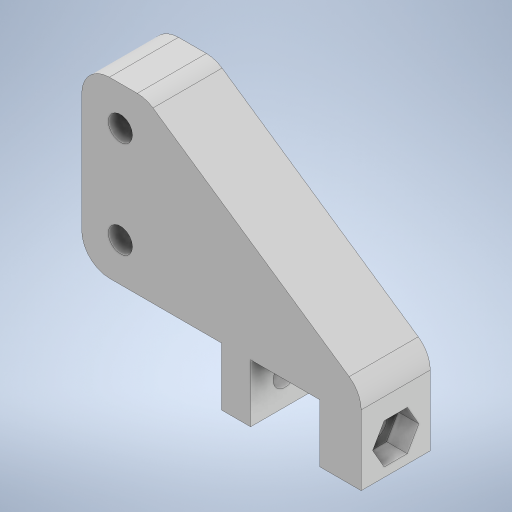
# Autodesk Inventor part: ClawShoulder
Saved by Autodesk Inventor 2023 (Build 270158000, 158)
## iProperties
Created: 2023-06-03
Part Number: ClawShoulder
Material: Ogólny
Document SubType Name: Modeling
Designer: Kamil
Density: 1 g/cm^3
Appearance: Domyślna
Author: Kamil
Autodesk Inventor part; units mm, degrees
ref_plane "YZ Plane" through (0, 0, 0) normal (1, 0, 0) x (0, 1, 0)
ref_plane "XZ Plane" through (0, 0, 0) normal (0, 1, 0) x (-1, 0, 0)
ref_plane "XY Plane" through (0, 0, 0) normal (0, 0, 1) x (1, 0, 0)
sketch "Szkic1" plane through (0, 0, 0) normal (0, 0, 1) x (1, 0, 0)
  line L0 (0.0002, 14.0002) -> (0.0002, 0.0002)
  line L1 (7.56, 19.5982) -> (5.6, 19.5982)
  line L2 (38.64, -14) -> (38.64, -5.6)
  line L3 (34.44, -14) -> (38.64, -14)
  line L4 (34.44, -5.6) -> (34.44, -14)
  line L5 (24.44, -14) -> (24.44, -5.6)
  line L6 (20.24, -14) -> (24.44, -14)
  line L7 (20.24, -5.6) -> (20.24, -14)
  circle A0 centre (5.6, 13.9982) radius 1.75
  circle A1 centre (5.6002, 0) radius 1.75
  line L8 (5.6, -5.6) -> (20.24, -5.6)
  line L9 (24.44, -5.6) -> (34.44, -5.6)
  line L10 (0, 19.5982) -> (9.2883, 19.5982)
  line L11 (0, -5.6) -> (0, 19.5982)
  line L12 (9.2883, 19.5982) -> (38.64, -0.5396)
  line L13 (38.64, -5.6) -> (38.64, -0.5396)
  line L14 (34.44, -5.6) -> (24.44, -5.6)
  line L15 (20.24, -5.6) -> (0, -5.6)
  point P0 (0, 0)
  point P1 (0, 14)
  point P2 (0, 0)
  dimension "d7" = 3.5
  dimension "d8" = 5.6
  dimension "d9" = 5.6
  dimension "d10" = 5.6
  dimension "d11" = 5.6
  dimension "d12" = 3.5
  constraints: 32 end point, 4 horizontal, 2 centre point, 2 parallel, 2 vertical, 1 other
  measures "d7" diameter of A0
  measures "d8" distance from line of L15 A1.centre
  measures "d9" distance from line of L11 A0.centre
  measures "d10" distance from line of L10 A0.centre
  measures "d11" distance from line of L0 A1.centre
  measures "d12" diameter of A1
extrude "Wyciągnięcie proste1" add sketch "Szkic1" against normal blind 10
sketch "Szkic2" plane through (20.24, -14, 0) normal (-1, 0, 0) x (0, 0, 1)
  line L0 (0, 8.4) -> (0, 0) projected
  line L1 (0, 8.4) -> (-10, 8.4) projected
  line L2 (-10, 0) -> (-10, 8.4) projected
  line L3 (0, 0) -> (-10, 0) projected
  line L4 (0, 0) -> (-10, 0) projected
  line L5 (-5, 0) -> (-5, 4.2)
  line L6 (-5, 4.2) -> (0, 4.2)
  circle A0 centre (-5, 4.2) radius 1.75
  point P0 (0, 14)
  dimension "d3" = 4.2
  dimension "d4" = 3.5
  constraints: 4 end point, 2 midpoint, 1 centre point, 1 coincident, 1 point on line, 1 vertical
  measures "d3" distance of L5.start L5.end
  measures "d4" diameter of A0
extrude "Wyciągnięcie proste2" cut sketch "Szkic2" against normal through all contours A0 L5 L6 | L6 L5 A0
move faces "Przesuń1" translate (1.8, 0, 0) faces at (38.64, -3.0473, -4.9297)
sketch "Szkic3" plane through (40.44, -14, 0) normal (1, 0, 0) x (0, 0, -1)
  circle A0 centre (5, 4.2) radius 1.75 projected
  circle A1 centre (5, 4.2) radius 2.9
  line L0 (3.3257, 1.3) -> (1.6514, 4.2)
  line L1 (1.6514, 4.2) -> (3.3257, 7.1)
  line L2 (3.3257, 7.1) -> (6.6743, 7.1)
  line L3 (6.6743, 7.1) -> (8.3486, 4.2)
  line L4 (8.3486, 4.2) -> (6.6743, 1.3)
  line L5 (6.6743, 1.3) -> (3.3257, 1.3)
  point P0 (0, 14)
  point P1 (5, 1.3)
  dimension "d16" = 5.8
  constraints: 12 end point, 2 coincident, 1 midpoint, 1 vertical alignment, 15 other
extrude "Wyciągnięcie proste3" cut sketch "Szkic3" against normal blind 3 contours A0 | A1 | A1 L3 L4 | A1 L2 L3 | L4 L5 A1 | A1 L1 L2 | L5 L0 A1 | A1 L0 L1
fillet "Zaokrąglenie2" radius 4 4 edges at (0, 19.5982, -5) (9.2883, 19.5982, -5) (40.44, -1.7745, -5) (0, -5.6, -5)
